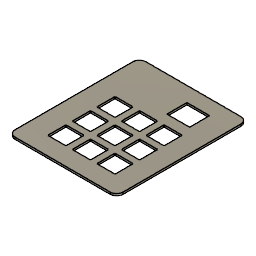
3x3Top (Autodesk Fusion 360 design; units mm, degrees)
part number: 2025-10-29-17-49-48-745
Autodesk Fusion 360 part; units mm, degrees
sketch "Szkic1" plane through (0, 0, 0) normal (0, 0, 1) x (1, 0, 0)
  line L0 (-13.996, 32.922) -> (69.916, 32.922)
  line L1 (69.916, 32.922) -> (69.916, -68.678)
  line L2 (69.916, -68.678) -> (-13.996, -68.678)
  line L3 (-13.996, -68.678) -> (-13.996, 32.922)
  line L4 (3.025, -2.525) -> (16.025, -2.525)
  line L5 (3.025, -16.525) -> (16.025, -16.525)
  line L6 (2.525, -3.025) -> (2.525, -16.025)
  line L7 (16.525, -3.025) -> (16.525, -16.025)
  arc A0 (3.025, -2.525) -> (2.525, -3.025) centre (3.025, -3.025) ccw
  arc A1 (16.525, -3.025) -> (16.025, -2.525) centre (16.025, -3.025) ccw
  arc A2 (2.525, -16.025) -> (3.025, -16.525) centre (3.025, -16.025) ccw
  arc A3 (16.025, -16.525) -> (16.525, -16.025) centre (16.025, -16.025) ccw
  line L8 (22.075, -2.525) -> (35.075, -2.525)
  line L9 (22.075, -16.525) -> (35.075, -16.525)
  line L10 (21.575, -3.025) -> (21.575, -16.025)
  line L11 (35.575, -3.025) -> (35.575, -16.025)
  arc A4 (22.075, -2.525) -> (21.575, -3.025) centre (22.075, -3.025) ccw
  arc A5 (35.575, -3.025) -> (35.075, -2.525) centre (35.075, -3.025) ccw
  arc A6 (21.575, -16.025) -> (22.075, -16.525) centre (22.075, -16.025) ccw
  arc A7 (35.075, -16.525) -> (35.575, -16.025) centre (35.075, -16.025) ccw
  line L12 (41.125, -2.525) -> (54.125, -2.525)
  line L13 (41.125, -16.525) -> (54.125, -16.525)
  line L14 (40.625, -3.025) -> (40.625, -16.025)
  line L15 (54.625, -3.025) -> (54.625, -16.025)
  arc A8 (41.125, -2.525) -> (40.625, -3.025) centre (41.125, -3.025) ccw
  arc A9 (54.625, -3.025) -> (54.125, -2.525) centre (54.125, -3.025) ccw
  arc A10 (40.625, -16.025) -> (41.125, -16.525) centre (41.125, -16.025) ccw
  arc A11 (54.125, -16.525) -> (54.625, -16.025) centre (54.125, -16.025) ccw
  line L16 (3.025, -21.575) -> (16.025, -21.575)
  line L17 (3.025, -35.575) -> (16.025, -35.575)
  line L18 (2.525, -22.075) -> (2.525, -35.075)
  line L19 (16.525, -22.075) -> (16.525, -35.075)
  arc A12 (3.025, -21.575) -> (2.525, -22.075) centre (3.025, -22.075) ccw
  arc A13 (16.525, -22.075) -> (16.025, -21.575) centre (16.025, -22.075) ccw
  arc A14 (2.525, -35.075) -> (3.025, -35.575) centre (3.025, -35.075) ccw
  arc A15 (16.025, -35.575) -> (16.525, -35.075) centre (16.025, -35.075) ccw
  line L20 (22.075, -21.575) -> (35.075, -21.575)
  line L21 (22.075, -35.575) -> (35.075, -35.575)
  line L22 (21.575, -22.075) -> (21.575, -35.075)
  line L23 (35.575, -22.075) -> (35.575, -35.075)
  arc A16 (22.075, -21.575) -> (21.575, -22.075) centre (22.075, -22.075) ccw
  arc A17 (35.575, -22.075) -> (35.075, -21.575) centre (35.075, -22.075) ccw
  arc A18 (21.575, -35.075) -> (22.075, -35.575) centre (22.075, -35.075) ccw
  arc A19 (35.075, -35.575) -> (35.575, -35.075) centre (35.075, -35.075) ccw
  line L24 (41.125, -21.575) -> (54.125, -21.575)
  line L25 (41.125, -35.575) -> (54.125, -35.575)
  line L26 (40.625, -22.075) -> (40.625, -35.075)
  line L27 (54.625, -22.075) -> (54.625, -35.075)
  arc A20 (41.125, -21.575) -> (40.625, -22.075) centre (41.125, -22.075) ccw
  arc A21 (54.625, -22.075) -> (54.125, -21.575) centre (54.125, -22.075) ccw
  arc A22 (40.625, -35.075) -> (41.125, -35.575) centre (41.125, -35.075) ccw
  arc A23 (54.125, -35.575) -> (54.625, -35.075) centre (54.125, -35.075) ccw
  line L28 (3.025, -40.625) -> (16.025, -40.625)
  line L29 (3.025, -54.625) -> (16.025, -54.625)
  line L30 (2.525, -41.125) -> (2.525, -54.125)
  line L31 (16.525, -41.125) -> (16.525, -54.125)
  arc A24 (3.025, -40.625) -> (2.525, -41.125) centre (3.025, -41.125) ccw
  arc A25 (16.525, -41.125) -> (16.025, -40.625) centre (16.025, -41.125) ccw
  arc A26 (2.525, -54.125) -> (3.025, -54.625) centre (3.025, -54.125) ccw
  arc A27 (16.025, -54.625) -> (16.525, -54.125) centre (16.025, -54.125) ccw
  line L32 (22.075, -40.625) -> (35.075, -40.625)
  line L33 (22.075, -54.625) -> (35.075, -54.625)
  line L34 (21.575, -41.125) -> (21.575, -54.125)
  line L35 (35.575, -41.125) -> (35.575, -54.125)
  arc A28 (22.075, -40.625) -> (21.575, -41.125) centre (22.075, -41.125) ccw
  arc A29 (35.575, -41.125) -> (35.075, -40.625) centre (35.075, -41.125) ccw
  arc A30 (21.575, -54.125) -> (22.075, -54.625) centre (22.075, -54.125) ccw
  arc A31 (35.075, -54.625) -> (35.575, -54.125) centre (35.075, -54.125) ccw
  line L36 (41.125, -40.625) -> (54.125, -40.625)
  line L37 (41.125, -54.625) -> (54.125, -54.625)
  line L38 (40.625, -41.125) -> (40.625, -54.125)
  line L39 (54.625, -41.125) -> (54.625, -54.125)
  arc A32 (41.125, -40.625) -> (40.625, -41.125) centre (41.125, -41.125) ccw
  arc A33 (54.625, -41.125) -> (54.125, -40.625) centre (54.125, -41.125) ccw
  arc A34 (40.625, -54.125) -> (41.125, -54.625) centre (41.125, -54.125) ccw
  arc A35 (54.125, -54.625) -> (54.625, -54.125) centre (54.125, -54.125) ccw
  line L40 (34.533, 21.279) -> (52.033, 21.279)
  line L41 (52.033, 21.279) -> (52.033, 5.879)
  line L42 (52.033, 5.879) -> (34.533, 5.879)
  line L43 (34.533, 5.879) -> (34.533, 21.279)
  dimension "d1" = 16.521
  dimension "d2" = 14.053
  dimension "d3" = 83.912
  dimension "d4" = 101.6
  dimension "d5" = 17.5
  dimension "d6" = 15.4
  dimension "d7" = 8.404
  dimension "d8" = 17.883
  constraint horizontal L0
  constraint vertical L1
  constraint horizontal L2
  constraint vertical L3
  constraint horizontal L40
  constraint vertical L41
  constraint horizontal L42
  constraint vertical L43
  measures "d1" distance of L3 L30
  measures "d2" distance of L2 L33
  measures "d3" distance of L0.start L0.end
  measures "d4" distance of L0.start L2.end
  measures "d5" distance of L40.start L40.end
  measures "d6" distance of L40.start L42.end
  measures "d7" distance of L12 L42
  measures "d8" distance of L1 L41
extrude "Wyciągnięcie proste1" add sketch "Szkic1" along normal blind 1.5
fillet "Zaokrąglenie1" radius 5 4 edges at (69.916, -68.678, 0.75) (-13.996, -68.678, 0.75) (-13.996, 32.922, 0.75) (69.916, 32.922, 0.75)
